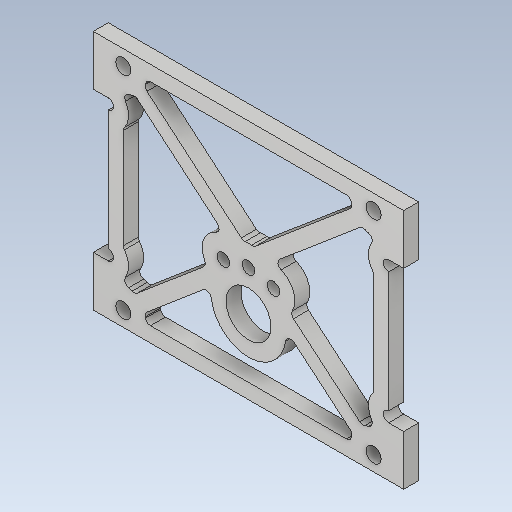
# Autodesk Inventor part: 横回転フレーム
Saved by Autodesk Inventor 2020 (Build 240168000, 168)
## iProperties
Created: 2019-09-04
Part Number: 横回転フレーム
Material: アルミニウム 2014-T4
Document SubType Name: Modeling
Designer: tanjihayato
Density: 2.8 g/cm^3
Appearance: サテン
Mass: 10.2156 g
Surface Area: 45.281 cm^2
Volume: 3.64842 cm^3
Author: tanjihayato
Autodesk Inventor part; units mm, degrees
note: some values were not read from the file. Chosen so that the rebuilt part matches the saved one: sketch regions of "押し出し3".
ref_plane "YZ Plane" through (0, 0, 0) normal (1, 0, 0) x (0, 1, 0)
ref_plane "XZ Plane" through (0, 0, 0) normal (0, 1, 0) x (-1, 0, 0)
ref_plane "XY Plane" through (0, 0, 0) normal (0, 0, 1) x (1, 0, 0)
sketch "スケッチ1" plane through (0, 0, 0) normal (0, 0, 1) x (1, 0, 0)
  line L0 (0, 0) -> (0, 4) construction
  line L1 (0, 0) -> (-5.3121, 14.0279)
  line L2 (-5.3121, 14.0279) -> (3.582, -2.7619)
  circle A0 centre (0.3052, 3.4238) radius 4
  line L3 (-57.3278, -140) -> (69.8706, -140)
  line L4 (0.3052, 3.4238) -> (-114.5721, -57.4302)
  circle A1 centre (0, 0) radius 23.1
  circle A2 centre (0, -29.1039) radius 6.0039
  line L5 (0, 0) -> (0, -29.1039) construction
  circle A3 centre (0, -29.1039) radius 20.05
  circle A4 centre (0, -4.0039) radius 5.05
  circle A5 centre (0, 4) radius 3
  circle A6 centre (0, -4.0039) radius 20.05
  circle A7 centre (-14, 13.4079) radius 2.2921
  circle A8 centre (14, 13.4079) radius 2.2921
  circle A9 centre (14, -21.4157) radius 2.2921
  circle A10 centre (-14, -21.4157) radius 2.2921
  circle A11 centre (-14, 13.4079) radius 14
  circle A12 centre (14, 13.4079) radius 14
  circle A13 centre (14, -21.4157) radius 14
  circle A14 centre (-14, -21.4157) radius 14
  line L6 (-14, 13.4079) -> (-14, -21.4157) construction
  line L7 (-14, -21.4157) -> (14, -21.4157) construction
  circle A15 centre (0, 0) radius 9
  line L8 (3.582, -2.7619) -> (-0.1629, 4.3075) construction
  line L9 (6.2551, -1.3458) -> (2.5102, 5.7235)
  line L10 (-2.836, 2.8915) -> (0.9089, -4.1779)
  arc A16 (0.9089, -4.1779) -> (6.2551, -1.3458) centre (3.582, -2.7619) ccw
  arc A17 (2.5102, 5.7235) -> (-2.836, 2.8915) centre (-0.1629, 4.3075) ccw
  line L11 (-5, 2.8868) -> (5, 2.8868) construction
  line L12 (5, 2.8868) -> (0, -5.7735) construction
  line L13 (0, -5.7735) -> (-5, 2.8868) construction
  circle A18 centre (-5, 2.8868) radius 1.5
  circle A19 centre (5, 2.8868) radius 1.5
  circle A20 centre (0, -5.7735) radius 1.5
  line L14 (-28, 26.018) -> (-28, -39.908)
  line L15 (28, 26.019) -> (28, -39.909)
  line L16 (-28, 29.3694) -> (28, 29.3694)
  circle A21 centre (0, 0) radius 25.1
  line L17 (-28, -18.848) -> (28, -18.848)
  circle A22 centre (0, -29.1039) radius 8.0039
  circle A23 centre (-25, 26.3694) radius 3
  circle A24 centre (25, 26.3694) radius 3
  circle A25 centre (25, -34.3772) radius 3
  circle A26 centre (-25, -34.3772) radius 3
  circle A27 centre (-25, -15.848) radius 3
  circle A28 centre (25, -15.848) radius 3
  circle A29 centre (-25, -15.848) radius 4.5
  circle A30 centre (25, -15.848) radius 4.5
  circle A31 centre (0, -4.0039) radius 4.5
  point P0 (1.7095, 0.7728)
  dimension "d0" = 4
  dimension "d1" = 15
  dimension "d2" = 11.348
  dimension "d3" = 19
  dimension "d4" = 8
  dimension "d5" = 12
  dimension "d6" = 140
  dimension "d7" = 130
  dimension "d8" = 46.2
  dimension "d9" = 29.1039
  dimension "d10" = 40.1
  dimension "d11" = 10.1
  dimension "d12" = 6
  dimension "d13" = 40.1
  dimension "d14" = 22.3421
  dimension "d15" = 22.3421
  dimension "d16" = 22.3421
  dimension "d17" = 22.3421
  dimension "d18" = 28
  dimension "d19" = 28
  dimension "d20" = 28
  dimension "d21" = 28
  dimension "d22" = 18
  dimension "d23" = 8
  dimension "d24" = 6.05
  dimension "d25" = 3
  dimension "d26" = 3
  dimension "d27" = 3
  dimension "d28" = 10
  dimension "d29" = 2
  dimension "d30" = 2
  dimension "d31" = 6
  dimension "d32" = 6
  dimension "d33" = 6
  dimension "d34" = 6
  dimension "d35" = 6
  dimension "d36" = 6
  dimension "d37" = 9
  dimension "d38" = 9
  dimension "d39" = 9
  constraints: 38 end point, 32 centre point, 28 tangent, 16 coincident, 8 point on line, 5 vertical, 4 point on circle, 3 horizontal, 3 perpendicular, 1 midpoint, 1 parallel, 7 other
  measures "d0" distance of L0.start L0.end
  measures "d1" distance of L0.start L1.end
  measures "d2" distance of L0.end L1.end
  measures "d3" distance of L1.end L2.end
  measures "d4" diameter of A0
  measures "d5" distance of L1.end L4.start
  measures "d6" distance from line of L3 L0.start
  measures "d7" distance of L4.start L4.end
  measures "d8" diameter of A1
  measures "d9" distance of L5.end L0.start
  measures "d10" diameter of A3
  measures "d11" diameter of A4
  measures "d12" diameter of A5
  measures "d13" diameter of A6
  measures "d14" distance of A7.centre A6.centre
  measures "d15" distance of A4.centre A8.centre
  measures "d16" distance of A4.centre A9.centre
  measures "d17" distance of A4.centre A10.centre
  measures "d18" diameter of A11
  measures "d19" diameter of A12
  measures "d20" diameter of A13
  measures "d21" diameter of A14
  measures "d22" diameter of A15
  measures "d23" distance of L2.end L8.end
  measures "d24" diameter of A17
  measures "d25" diameter of A18
  measures "d26" diameter of A19
  measures "d27" diameter of A20
  measures "d28" distance of L11.end L12.end
  measures "d29" radial gap between concentric circles of A1 A21
  measures "d30" radial gap between concentric circles of A2 A22
  measures "d31" diameter of A23
  measures "d32" diameter of A24
  measures "d33" diameter of A25
  measures "d34" diameter of A26
  measures "d35" diameter of A27
  measures "d36" diameter of A28
  measures "d37" diameter of A29
  measures "d38" diameter of A30
  measures "d39" diameter of A31
sketch "スケッチ2" plane through (0, 0, 0) normal (0, 0, 1) x (1, 0, 0)
  circle A0 centre (-25, 26.3694) radius 3 construction
  circle A1 centre (25, 26.3694) radius 3 construction
  circle A2 centre (25, -15.848) radius 3 construction
  circle A3 centre (-25, -15.848) radius 3 construction
  circle A4 centre (5, 2.8868) radius 1.5 construction
  circle A5 centre (-5, 2.8868) radius 1.5 construction
  circle A6 centre (0, 4) radius 3 construction
  circle A7 centre (-25, 26.3694) radius 1.5
  circle A8 centre (25, 26.3694) radius 1.5
  circle A9 centre (25, -15.848) radius 1.5
  circle A10 centre (-25, -15.848) radius 1.5
  line L0 (-31, 29.3694) -> (31, 29.3694)
  line L1 (31, 29.3694) -> (31, 19.3694)
  line L2 (31, 19.3694) -> (28, 19.3694)
  line L3 (28, 17.2694) -> (28, -6.748)
  line L4 (28, -8.848) -> (31, -8.848)
  line L5 (31, -8.848) -> (31, -18.848)
  line L6 (31, -18.848) -> (-31, -18.848)
  line L7 (-31, -18.848) -> (-31, -8.848)
  line L8 (-31, -8.848) -> (-28, -8.848)
  line L9 (-28, -6.748) -> (-28, 17.2694)
  line L10 (-28, 19.3694) -> (-31, 19.3694)
  line L11 (-31, 19.3694) -> (-31, 29.3694)
  circle A11 centre (-5, 2.8868) radius 1.25
  circle A12 centre (5, 2.8868) radius 1.25
  circle A13 centre (0, 4) radius 1.25
  circle A14 centre (0, -4.0039) radius 4.5 projected
  arc A15 (-28, 17.2694) -> (-28, 19.3694) centre (-28, 18.3194) ccw
  arc A16 (-28, -8.848) -> (-28, -6.748) centre (-28, -7.798) ccw
  arc A17 (28, 19.3694) -> (28, 17.2694) centre (28, 18.3194) ccw
  arc A18 (28, -6.748) -> (28, -8.848) centre (28, -7.798) ccw
  arc A19 (-6.8462, -0.9413) -> (6.8462, -0.9413) centre (0, -4.0039) ccw
  arc A20 (6.8462, -0.9413) -> (3.2371, 6.7539) centre (5, 2.8868) ccw
  arc A21 (3.2371, 6.7539) -> (-3.2371, 6.7539) centre (0, 4) ccw
  arc A22 (-3.2371, 6.7539) -> (-6.8462, -0.9413) centre (-5, 2.8868) ccw
  arc A23 (-20.5, -15.848) -> (-23.962, -11.4694) centre (-25, -15.848) ccw
  arc A24 (-23.962, 21.9907) -> (-20.5, 26.3694) centre (-25, 26.3694) ccw
  arc A25 (-25, 15.5986) -> (-24.5766, 20.4834) centre (-28, 18.3194) ccw
  line L12 (-25, 15.5986) -> (-25, -5.0773)
  arc A26 (-24.5766, -9.962) -> (-25, -5.0773) centre (-28, -7.798) ccw
  arc A27 (25, -5.0773) -> (24.5766, -9.962) centre (28, -7.798) ccw
  line L13 (25, -5.0773) -> (25, 15.5986)
  arc A28 (24.5766, 20.4834) -> (25, 15.5986) centre (28, 18.3194) ccw
  line L14 (20.5, 26.3694) -> (-20.5, 26.3694)
  arc A29 (-23.962, 21.9907) -> (-24.5766, 20.4834) centre (-23.7313, 21.0177) ccw
  arc A30 (-24.5766, -9.962) -> (-23.962, -11.4694) centre (-23.7313, -10.4963) ccw
  arc A31 (23.962, -11.4694) -> (24.5766, -9.962) centre (23.7313, -10.4963) ccw
  arc A32 (24.5766, 20.4834) -> (23.962, 21.9907) centre (23.7313, 21.0177) ccw
  arc A33 (23.962, -11.4694) -> (20.5, -15.848) centre (25, -15.848) ccw
  line L15 (-20.5, -15.848) -> (20.5, -15.848)
  arc A34 (20.5, 26.3694) -> (23.962, 21.9907) centre (25, 26.3694) ccw
  line L16 (-25, 26.3694) -> (25, -15.848) construction
  line L17 (-25.9677, 25.2233) -> (24.0323, -16.9941)
  line L18 (25.9677, -14.7019) -> (-24.0323, 27.5155)
  arc A35 (-24.0323, 27.5155) -> (-25.9677, 25.2233) centre (-25, 26.3694) ccw
  arc A36 (24.0323, -16.9941) -> (25.9677, -14.7019) centre (25, -15.848) ccw
  line L19 (25, 26.3694) -> (-25, -15.848) construction
  line L20 (24.0323, 27.5155) -> (-25.9677, -14.7019)
  line L21 (-24.0323, -16.9941) -> (25.9677, 25.2233)
  arc A37 (25.9677, 25.2233) -> (24.0323, 27.5155) centre (25, 26.3694) ccw
  arc A38 (-25.9677, -14.7019) -> (-24.0323, -16.9941) centre (-25, -15.848) ccw
  point P0 (0, 0)
  point P1 (0, 5.2607)
  point P2 (0, 5.2607)
  dimension "d40" = 3
  dimension "d41" = 3
  dimension "d42" = 3
  dimension "d43" = 3
  dimension "d44" = 10
  dimension "d45" = 3
  dimension "d46" = 3
  dimension "d47" = 10
  dimension "d48" = 10
  dimension "d49" = 3
  dimension "d50" = 3
  dimension "d51" = 10
  dimension "d52" = 2.5
  dimension "d53" = 2.5
  dimension "d54" = 2.5
  dimension "d57" = 2.1
  dimension "d58" = 2.1
  dimension "d59" = 2.1
  dimension "d60" = 2.1
  dimension "d63" = 3
  dimension "d64" = 3
  dimension "d65" = 3
  dimension "d66" = 3
  dimension "d68" = 3
  dimension "d69" = 3
  dimension "d72" = 2
  dimension "d73" = 3
  dimension "d74" = 2
  dimension "d75" = 2
  dimension "d76" = 2
  dimension "d77" = 3
  dimension "d78" = 3
  dimension "d79" = 4.05
  dimension "d81" = 3
  dimension "d82" = 4.5
  dimension "d83" = 4.05
  dimension "d84" = 3
  dimension "d85" = 4.5
  dimension "d86" = 4.05
  dimension "d87" = 3
  dimension "d88" = 3
  constraints: 48 end point, 48 point on circle, 31 centre point, 24 tangent, 8 point on line, 7 coincident, 6 perpendicular, 2 concentric, 2 horizontal, 2 midpoint, 2 parallel
  measures "d40" diameter of A7
  measures "d41" diameter of A8
  measures "d42" diameter of A9
  measures "d43" diameter of A10
  measures "d44" distance of L0.end L1.end
  measures "d45" distance of L1.end L2.end
  measures "d46" distance of L4.start L4.end
  measures "d47" distance of L4.end L5.end
  measures "d48" distance of L6.end L7.end
  measures "d49" distance of L7.end L8.end
  measures "d50" distance of L10.start L10.end
  measures "d51" distance of L10.end L0.start
  measures "d52" diameter of A11
  measures "d53" diameter of A12
  measures "d54" diameter of A13
  measures "d57" diameter of A15
  measures "d58" diameter of A16
  measures "d59" diameter of A17
  measures "d60" diameter of A18
  measures "d63" radial gap between concentric circles of A14 A19
  measures "d64" radial gap between concentric circles of A12 A20
  measures "d65" radial gap between concentric circles of A13 A21
  measures "d66" radial gap between concentric circles of A11 A22
  measures "d68" radial gap between concentric circles of A10 A23
  measures "d69" radial gap between concentric circles of A7 A24
  measures "d72" diameter of A29
  measures "d73" radial gap between concentric circles of A25 A15
  measures "d74" diameter of A30
  measures "d75" diameter of A31
  measures "d76" diameter of A32
  measures "d77" distance between parallel lines of L9 L12
  measures "d78" distance between parallel lines of L0 L14
  measures "d79" radius of A26
  measures "d81" distance between parallel lines of L3 L13
  measures "d82" radius of A34
  measures "d83" radius of A28
  measures "d84" distance between parallel lines of L6 L15
  measures "d85" radius of A33
  measures "d86" radius of A27
  measures "d87" diameter of A36
  measures "d88" diameter of A38
extrude "押し出し3" add sketch "スケッチ2" along normal blind 3 contours A7 L18 A24 L17 | L18 A21 A22 L17 A24 | L18 L20 L17 A22 A21 | A21 L20 L18 | L17 L20 A11 A22 | L20 A34 L21 A20 A21 | A21 A20 L21 L18 L20 | L18 L21 A13 L17 L20 | L20 A11 L17 A13 L21 A19 A22 | A22 A19 L21 A23 L20 | L20 A8 L21 A34 | L21 A20 L18 A12 | L18 A12 A20 A19 L17 A13 L21 | A23 L21 A10 L20 | L21 A13 L17 A19 | L18 A33 L17 A19 A20 | L18 A9 L17 A33 | L0 L1 L2 A17 L3 A18 L4 L5 L6 L7 L8 A16 L9 A15 L10 L11
extrude "押し出し4" cut sketch "スケッチ2" along normal blind 3 contours L20 A11 | A11 L20 | L17 L21 A13 | A13 L21 L17 | L18 A12 | A12 L18 | A13 L17 L21 | L21 L17 A13
fillet "フィレット1" radius 1 24 edges at (-20.7906, -14.257, 1.5) (-20.5, -15.848, 1.5) (20.5, -15.848, 1.5) (20.7906, -14.257, 1.5) (22.726, -11.9648, 1.5) (25, -5.0773, 1.5) (25, 15.5986, 1.5) (22.726, 22.4862, 1.5) (20.7906, 24.7784, 1.5) (20.5, 26.3694, 1.5) (-20.5, 26.3694, 1.5) (-20.7906, 24.7784, 1.5) (-22.726, 22.4862, 1.5) (-25, 15.5986, 1.5) (-25, -5.0773, 1.5) (-22.726, -11.9648, 1.5) (-7.4291, -2.9753, 1.5) (7.4291, -2.9753, 1.5) (8.3034, 0.2129, 1.5) (4.514, 7.1089, 1.5) (1.0571, 8.1164, 1.5) (-1.0571, 8.1164, 1.5) (-4.514, 7.1089, 1.5) (-8.3034, 0.2129, 1.5)
equation "\"d15\" = d14"
equation "\"d16\" = d14"
equation "\"d17\" = d14"
